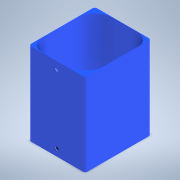
# Autodesk Inventor part: Storage_tank
Saved by Autodesk Inventor 2020 (Build 240168000, 168)
## iProperties
Created: 2020-08-16
Part Number: Storage_tank
Material: Generic
Document SubType Name: Modeling
Designer: Abbas
Density: 1 g/cm^3
Appearance: Default
Author: Abbas
Autodesk Inventor part; units mm, degrees
ref_plane "YZ Plane" through (0, 0, 0) normal (1, 0, 0) x (0, 1, 0)
ref_plane "XZ Plane" through (0, 0, 0) normal (0, 1, 0) x (-1, 0, 0)
ref_plane "XY Plane" through (0, 0, 0) normal (0, 0, 1) x (1, 0, 0)
sketch "Sketch1" plane through (0, 0, 0) normal (0, 1, 0) x (-1, 0, 0)
  line L0 (235, 275) -> (-235, 275)
  line L1 (-235, 275) -> (-235, -275)
  line L2 (-235, -275) -> (235, -275)
  line L3 (235, -275) -> (235, 275)
  line L4 (235, 275) -> (-235, -275) construction
  line L5 (-235, 275) -> (235, -275) construction
  line L6 (232, 272) -> (-232, 272)
  line L7 (-232, 272) -> (-232, -272)
  line L8 (-232, -272) -> (232, -272)
  line L9 (232, -272) -> (232, 272)
  point P0 (0, 0)
  dimension "d0" = 470
  dimension "d1" = 550
  dimension "d2" = 3
  constraints: 20 end point, 4 parallel, 2 midpoint, 2 perpendicular, 1 horizontal, 3 other
  measures "d0" distance of L2.end L1.end
  measures "d1" distance of L1.end L0.end
  measures "d2" distance between parallel lines of L3 L9
extrude "Extrusion1" add sketch "Sketch1" along normal blind 3 contours L9 L8 L7 L6
extrude "Extrusion2" add sketch "Sketch1" along normal blind 690
fillet "Fillet1" radius 106 1 edges at (-232, 346.5, 272)
fillet "Fillet2" radius 148 1 edges at (-232, 346.5, -272)
fillet "Fillet3" radius 164 1 edges at (232, 346.5, 272)
fillet "Fillet4" radius 105 1 edges at (232, 346.5, -272)
fillet "Fillet5" radius 20 4 edges at (235, 345, 275) (235, 345, -275) (-235, 345, 275) (-235, 345, -275)
sketch "Sketch2" plane through (-215, 0, 275) normal (0, 0, 1) x (1, 0, 0)
  line L0 (0, 0) -> (0, 690) projected
  line L1 (0, 690) -> (430, 690) projected
  line L2 (0, 0) -> (430, 0) projected
  point P0 (215, 0)
  point P1 (215, 630)
  point P2 (215, 60)
  dimension "d19" = 215
  dimension "d20" = 60
  dimension "d21" = 215
  dimension "d22" = 60
  measures "d19" distance from line of L0 point (215, 630)
  measures "d20" distance from line of L1 point (215, 630)
  measures "d21" distance from line of L0 point (215, 60)
  measures "d22" distance from line of L2 point (215, 60)
hole "Hole1" at (0, 630, 275) at (0, 60, 275) direction (0, 0, -1) diameter 25.4 depth 26 tip angle 118
body "Solid1"
